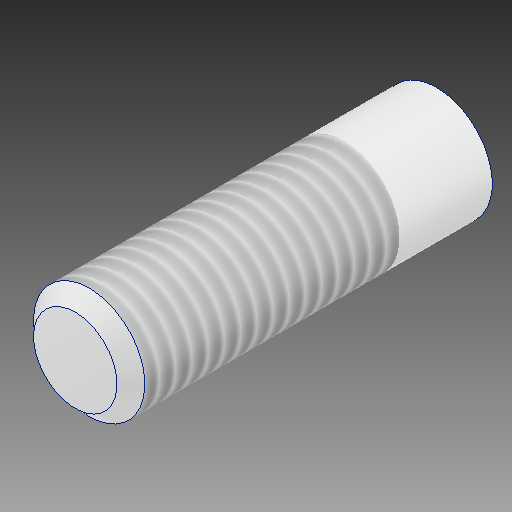
# Autodesk Inventor part: Spindle Iso M12 Setscrew
Saved by Autodesk Inventor 2021.3 (Build 253353000, 353)
## iProperties
Created: 2021-04-22
Part Number: Spindle Iso M12 Setscrew
Material: Aluminum 6061
Document SubType Name: Modeling
Designer: domin
Density: 2.7 g/cm^3
Appearance: Aluminum - Flat
Author: domin
Autodesk Inventor part; units mm, degrees
ref_plane "YZ Plane" through (0, 0, 0) normal (1, 0, 0) x (0, 1, 0)
ref_plane "XZ Plane" through (0, 0, 0) normal (0, 1, 0) x (-1, 0, 0)
ref_plane "XY Plane" through (0, 0, 0) normal (0, 0, 1) x (1, 0, 0)
sketch "Sketch3" plane through (0, 0, 0) normal (1, 0, 0) x (0, 1, 0)
  line L0 (6, 19.5) -> (0, 19.5)
  line L1 (0, 19.5) -> (0, -19.5)
  line L2 (0, -19.5) -> (6, -19.5)
  line L3 (6, -19.5) -> (6, 19.5)
  point P0 (0, 0)
  dimension "d11" = 39
  dimension "d12" = 0
  dimension "d13" = 6
  dimension "d15" = 19.5
  constraints: 8 end point, 2 parallel, 1 horizontal, 1 perpendicular
  measures "d11" distance between parallel lines of L2 L0
  measures "d12" distance from line of point (0, 0) L1
  measures "d13" distance between parallel lines of L1 L3
  measures "d15" distance from line of point (0, 0) L0
revolve "Revolution2" add sketch "Sketch3" angle 360 about axis through (0, 0, 19.5) along (0, 0, -1)
sketch "Sketch6" plane through (0, 0, -19.5) normal (0, 0, -1) x (-1, 0, 0)
  circle A0 centre (0, 0) radius 2.5
  dimension "d39" = 5
  constraints: 1 centre point, 1 coincident
  measures "d39" diameter of A0
hole "Hole3" at (0, 0, -19.5) direction (0, 0, 1) diameter 5 depth 14 tip angle 118
sketch "Sketch7" plane through (0, 0, 0) normal (0, 1, 0) x (-1, 0, 0)
  circle A0 centre (0, -14.5) radius 2
  line L0 (-6, -19.5) -> (6, -19.5) projected
  point P0 (0, 0)
  dimension "d47" = 4
  dimension "d49" = 5
  constraints: 1 centre point, 1 vertical alignment
  measures "d47" diameter of A0
  measures "d49" distance from line of L0 A0.centre
hole "Hole4" at (0, 0, -14.5) direction (0, -1, 0) diameter 3.242 end through all thread size "M4x0.7" class "6H" standard "ISO Metric profile"
thread "Thread2" size "M12x1.75" class "6g" standard "ANSI Metric M Profile" length 29
chamfer "Chamfer3" distance 1.5 angle 45 1 edges at (0, -6, 19.5)
equation "\"d15\" = 0.5 * d11"
equation "\"d40\" = d39"
body "Solid2"
